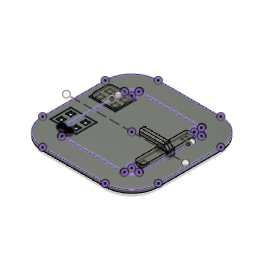
door v4 (Autodesk Fusion 360 design; units mm, degrees)
Autodesk Fusion 360 part; units mm, degrees
sketch "plate" plane through (0, 0, 0) normal (0, 1, 0) x (1, 0, 0)
  line L0 (20, -25) -> (-20, -25)
  line L1 (-25, -20) -> (-25, 20)
  line L2 (-20, 25) -> (20, 25)
  line L3 (25, 20) -> (25, -20)
  line L4 (25, -25) -> (-25, 25) construction
  line L5 (-25, -25) -> (25, 25) construction
  arc A0 (-20, 25) -> (-25, 20) centre (-20, 20) ccw
  arc A1 (-25, -20) -> (-20, -25) centre (-20, -20) ccw
  arc A2 (20, -25) -> (25, -20) centre (20, -20) ccw
  arc A3 (25, 20) -> (20, 25) centre (20, 20) ccw
  line L6 (20, -37) -> (-20, -37)
  arc A4 (-37, -20) -> (-20, -37) centre (-20, -20) ccw
  line L7 (-37, -20) -> (-37, 20)
  arc A5 (-20, 37) -> (-37, 20) centre (-20, 20) ccw
  line L8 (-20, 37) -> (20, 37)
  arc A6 (37, 20) -> (20, 37) centre (20, 20) ccw
  line L9 (37, 20) -> (37, -20)
  arc A7 (20, -37) -> (37, -20) centre (20, -20) ccw
  arc A8 (24.5, 20) -> (20, 24.5) centre (20, 20) ccw
  line L10 (-20, 24.5) -> (20, 24.5)
  arc A9 (-20, 24.5) -> (-24.5, 20) centre (-20, 20) ccw
  line L11 (-24.5, -20) -> (-24.5, 20)
  arc A10 (-24.5, -20) -> (-20, -24.5) centre (-20, -20) ccw
  line L12 (20, -24.5) -> (-20, -24.5)
  arc A11 (20, -24.5) -> (24.5, -20) centre (20, -20) ccw
  line L13 (24.5, 20) -> (24.5, -20)
  dimension "d1" = 50
  dimension "d2" = 50
  dimension "d3" = -12
  dimension "d4" = 5
  dimension "d5" = 0.5
  constraint horizontal L0
  constraint perpendicular L0 L1
  constraint parallel L0 L2
  constraint parallel L1 L3
  constraint coincident L4 origin
  constraint coincident L5 origin
  constraint coincident L4.end L2
  constraint coincident L4.end L1
  constraint tangent L2 A0
  constraint tangent L1 A0
  constraint coincident L5.start L1
  constraint coincident L5.start L0
  constraint tangent L1 A1
  constraint tangent L0 A1
  constraint equal A0 A1
  constraint coincident L4.start L0
  constraint coincident L4.start L3
  constraint tangent L0 A2
  constraint tangent L3 A2
  constraint equal A0 A2
  constraint coincident L5.end L3
  constraint coincident L5.end L2
  constraint tangent L3 A3
  constraint tangent L2 A3
  constraint equal A0 A3
  measures "d1" distance of L4.end L5.end
  measures "d2" distance of L5.start L4.end
  measures "d4" radius of A0
extrude "Extrude1" add sketch "plate" against normal blind 2 makes body 1 at (29, 0, -6.6667) makes body 2 at (-8.1667, 0, -9.6667)
sketch "hinge" plane through (0, 0, 0) normal (0, 1, 0) x (1, 0, 0)
  line L0 (-20, -25) -> (20, -25)
  arc A0 (-25, -20) -> (-20, -25) centre (-20, -20) ccw
  line L1 (-25, 20) -> (-25, -20)
  arc A1 (-20, 25) -> (-25, 20) centre (-20, 20) ccw
  line L2 (20, 25) -> (-20, 25)
  arc A2 (25, 20) -> (20, 25) centre (20, 20) ccw
  line L3 (25, -20) -> (25, 20)
  arc A3 (20, -25) -> (25, -20) centre (20, -20) ccw
  line L4 (20, -37) -> (-20, -37)
  arc A4 (20, -37) -> (37, -20) centre (20, -20) ccw
  line L5 (37, 20) -> (37, -20)
  arc A5 (37, 20) -> (20, 37) centre (20, 20) ccw
  line L6 (-20, 37) -> (20, 37)
  arc A6 (-20, 37) -> (-37, 20) centre (-20, 20) ccw
  line L7 (-37, -20) -> (-37, 20)
  arc A7 (-37, -20) -> (-20, -37) centre (-20, -20) ccw
  line L8 (-24.5, -20) -> (-24.5, 20)
  arc A8 (-24.5, -20) -> (-20, -24.5) centre (-20, -20) ccw
  line L9 (20, -24.5) -> (-20, -24.5)
  arc A9 (20, -24.5) -> (24.5, -20) centre (20, -20) ccw
  line L10 (24.5, 20) -> (24.5, -20)
  arc A10 (24.5, 20) -> (20, 24.5) centre (20, 20) ccw
  line L11 (-20, 24.5) -> (20, 24.5)
  arc A11 (-20, 24.5) -> (-24.5, 20) centre (-20, 20) ccw
  line L12 (-31, 17) -> (-28, 17)
  line L13 (-28, 17) -> (-28, 14)
  line L14 (-28, 14) -> (-31, 14)
  line L15 (-31, 14) -> (-31, 17)
  line L16 (-31, 11) -> (-28, 11)
  line L17 (-28, 11) -> (-28, 8)
  line L18 (-28, 8) -> (-31, 8)
  line L19 (-31, 8) -> (-31, 11)
  line L20 (0, 0) -> (-41.7851, 0) construction
  line L21 (-25, 11.8799) -> (-24.5, 11.8799) construction
  line L22 (-24.75, 11.8799) -> (-24.75, 16.1547) construction
  line L23 (-18.5, 17) -> (-21.5, 17)
  line L24 (-18.5, 14) -> (-18.5, 17)
  line L25 (-21.5, 17) -> (-21.5, 14)
  line L26 (-21.5, 14) -> (-18.5, 14)
  line L27 (-18.5, 11) -> (-21.5, 11)
  line L28 (-18.5, 8) -> (-18.5, 11)
  line L29 (-21.5, 11) -> (-21.5, 8)
  line L30 (-21.5, 8) -> (-18.5, 8)
  line L31 (-33, 19) -> (-16.5, 19)
  line L32 (-16.5, 19) -> (-16.5, 6)
  line L33 (-16.5, 6) -> (-33, 6)
  line L34 (-33, 6) -> (-33, 19)
  line L35 (-18.5, -11) -> (-21.5, -11)
  line L36 (-21.5, -8) -> (-18.5, -8)
  line L37 (-18.5, -17) -> (-21.5, -17)
  line L38 (-31, -8) -> (-31, -11)
  line L39 (-33, -6) -> (-33, -19)
  line L40 (-21.5, -11) -> (-21.5, -8)
  line L41 (-31, -17) -> (-28, -17)
  line L42 (-31, -11) -> (-28, -11)
  line L43 (-18.5, -14) -> (-18.5, -17)
  line L44 (-16.5, -19) -> (-16.5, -6)
  line L45 (-18.5, -8) -> (-18.5, -11)
  line L46 (-28, -17) -> (-28, -14)
  line L47 (-21.5, -17) -> (-21.5, -14)
  line L48 (-21.5, -14) -> (-18.5, -14)
  line L49 (-28, -14) -> (-31, -14)
  line L50 (-16.5, -6) -> (-33, -6)
  line L51 (-33, -19) -> (-16.5, -19)
  line L52 (-31, -14) -> (-31, -17)
  line L53 (-28, -8) -> (-31, -8)
  line L54 (-28, -11) -> (-28, -8)
  line L55 (19.75, 15) -> (22.75, 15)
  line L56 (22.75, 15) -> (22.75, 12)
  line L57 (22.75, 12) -> (19.75, 12)
  line L58 (19.75, 12) -> (19.75, 15)
  line L59 (24.5, 11.146) -> (25, 11.146) construction
  line L60 (24.75, 11.146) -> (24.75, 13.5187) construction
  line L61 (0, 0) -> (34.3439, 0) construction
  line L62 (18.25, 17) -> (24.25, 17)
  line L63 (24.25, 17) -> (24.25, 0)
  line L64 (24.25, 0) -> (18.25, 0)
  line L65 (18.25, 0) -> (18.25, 17)
  line L66 (22.75, -12) -> (19.75, -12)
  line L67 (19.75, -12) -> (19.75, -15)
  line L68 (19.75, -15) -> (22.75, -15)
  line L69 (22.75, -15) -> (22.75, -12)
  line L70 (18.25, -17) -> (24.25, -17)
  line L71 (24.25, -17) -> (24.25, 0)
  line L72 (18.25, 0) -> (18.25, -17)
  point P0 (-25, -20)
  point P1 (-20, -20)
  point P2 (-20, -20)
  point P3 (-24.5, -20)
  dimension "d8" = 3
  dimension "d9" = 3
  dimension "d10" = 3
  dimension "d11" = 3
  dimension "d12" = 3
  dimension "d13" = 3
  dimension "d14" = 8
  dimension "d15" = 2
  dimension "d16" = 2
  dimension "d17" = 2
  dimension "d18" = 2
  dimension "d29" = 3
  dimension "d30" = 3
  dimension "d31" = 2
  dimension "d32" = 12
  dimension "d33" = 1.5
  dimension "d34" = 2
  dimension "d35" = 1.5
  constraint horizontal L12
  constraint vertical L13
  constraint horizontal L14
  constraint vertical L15
  constraint horizontal L16
  constraint vertical L17
  constraint horizontal L18
  constraint vertical L19
  constraint coincident L20.start L61.start
  constraint perpendicular L7 L20
  constraint collinear L13 L17
  constraint coincident L1 L21.start
  constraint coincident L8 L21.end
  constraint perpendicular L8 L21
  constraint midpoint L21 L22.start
  constraint perpendicular L21 L22
  constraint symmetric L12.start L22 L23.start
  constraint symmetric L12.end L22 L23.end
  constraint symmetric L13.end L22 L25.end
  constraint symmetric L14.end L22 L24.start
  constraint symmetric L16.start L22 L27.start
  constraint symmetric L16.end L22 L27.end
  constraint symmetric L17.end L22 L29.end
  constraint symmetric L18.end L22 L28.start
  constraint horizontal L31
  constraint vertical L32
  constraint horizontal L33
  constraint vertical L34
  constraint symmetric L1.start L20 P0
  constraint symmetric A1.centre L20 P2
  constraint symmetric L8.end L20 P3
  constraint symmetric L12.start L20 L41.start
  constraint symmetric L12.end L20 L41.end
  constraint symmetric L13.end L20 L46.end
  constraint symmetric L14.end L20 L49.end
  constraint symmetric L16.start L20 L38.end
  constraint symmetric L16.end L20 L42.end
  constraint symmetric L17.end L20 L53.start
  constraint symmetric L18.end L20 L38.start
  constraint symmetric L20 L23.start L37.start
  constraint symmetric L20 L23.end L37.end
  constraint symmetric L20 L24.start L43.start
  constraint symmetric L20 L25.end L47.end
  constraint symmetric L20 L27.start L35.start
  constraint symmetric L20 L27.end L35.end
  constraint symmetric L20 L28.start L36.end
  constraint symmetric L20 L29.end L36.start
  constraint symmetric L20 L31.start L39.end
  constraint symmetric L20 L31.end L44.start
  constraint symmetric L20 L32.end L44.end
  constraint symmetric L20 L33.end L39.start
  constraint horizontal L55
  constraint vertical L56
  constraint horizontal L57
  constraint vertical L58
  constraint coincident L10 L59.start
  constraint coincident L3 L59.end
  constraint perpendicular L3 L59
  constraint midpoint L59 L60.start
  constraint perpendicular L59 L60
  constraint parallel L20 L61
  constraint horizontal L62
  constraint vertical L63
  constraint horizontal L64
  constraint vertical L65
  constraint collinear L61 L64
  constraint symmetric L55.start L61 L67.end
  constraint symmetric L55.end L61 L68.end
  constraint symmetric L56.end L61 L66.start
  constraint symmetric L57.end L61 L66.end
  constraint symmetric L61 L62.start L70.start
  constraint symmetric L61 L62.end L70.end
  constraint symmetric L61 L63.end L64.start
  constraint symmetric L61 L64.end L65.start
  measures "d8" distance of L12.start L12.end
  measures "d9" distance of L12.start L14.end
  measures "d10" distance of L16.start L16.end
  measures "d11" distance of L16.start L18.end
  measures "d12" distance of L14 L16
  measures "d13" distance of L1 L13
  measures "d14" distance of L18 L20
  measures "d15" distance of L24 L32
  measures "d16" distance of L23 L31
  measures "d17" distance of L30 L33
  measures "d18" distance of L15 L34
  measures "d29" distance of L55.start L55.end
  measures "d30" distance of L55.start L57.end
  measures "d31" distance of L56 L60
  measures "d32" distance of L57 L61
  measures "d33" distance of L58 L65
  measures "d34" distance of L55 L62
  measures "d35" distance of L56 L63
extrude "Extrude2" cut sketch "hinge" against normal blind 3 contours L12 L13 L14 L15 | L16 L17 L18 L19 | L23 L24 L25 L26 | L27 L28 L29 L30 | L35 L36 L40 L45 | L37 L43 L47 L48 | L38 L42 L53 L54 | L41 L46 L49 L52 bodies 1 2
extrude "Extrude3" add sketch "hinge" against normal blind 3 separate body contours L12 L13 L14 L15 | L16 L17 L18 L19 | L23 L24 L25 L26 | L27 L28 L29 L30 makes body 3 at (-21.5, -1, -16) makes body 4 at (-18.5, -1, -9) makes body 5 at (-28, -1, -16) makes body 6 at (-28, -1, -10)
extrude "Extrude4" add sketch "hinge" along normal blind 1 contours L1 L31 L33 L34 | L1 L8 L31 L33 | L8 L31 L32 L33 | L12 L13 L14 L15 | L16 L17 L18 L19 | L23 L24 L25 L26 | L27 L28 L29 L30 bodies 3 4 5 6
fillet "Fillet1" radius 3 4 edges at (-33, 0.5, -6) (-33, 0.5, -19) (-16.5, 0.5, -19) (-16.5, 0.5, -6) on bodies 3
chamfer "Chamfer1" distance 1.5 angle 45 1 edges at (24.5, -2, 0) tangent chain off on bodies 2
chamfer "Chamfer2" distance 1 angle 45 32 edges at (-28, -2, 15.5) (-29.5, -2, 14) (-31, -2, 15.5) (-29.5, -2, 17) (-28, -2, 9.5) (-29.5, -2, 8) (-31, -2, 9.5) (-29.5, -2, 11) (-28, -2, -9.5) (-29.5, -2, -8) (-29.5, -2, -11) (-31, -2, -9.5) (-28, -2, -15.5) (-29.5, -2, -14) (-29.5, -2, -17) (-31, -2, -15.5) (-18.5, -2, 15.5) (-20, -2, 17) (-21.5, -2, 15.5) (-20, -2, 14) (-20, -2, 8) (-21.5, -2, 9.5) (-20, -2, 11) (-18.5, -2, 9.5) (-18.5, -2, -9.5) (-20, -2, -11) (-20, -2, -8) (-21.5, -2, -9.5) (-18.5, -2, -15.5) (-20, -2, -17) (-21.5, -2, -15.5) (-20, -2, -14) tangent chain off on bodies 1 2
extrude "Extrude6" add sketch "hinge" against normal blind 3 separate body contours L55 L56 L57 L58 | L66 L67 L68 L69 makes body 7 at (20.75, -1, -15) makes body 8 at (22.75, -1, 14)
extrude "Extrude7" add sketch "hinge" along normal blind 2 contours L55 L56 L57 L58 | L62 L63 L64 L65 | L64 L70 L71 L72 | L66 L67 L68 L69 bodies 7 8
extrude "Extrude5" cut sketch "hinge" against normal blind 3 contours L55 L56 L57 L58 | L66 L67 L68 L69 bodies 2
fillet "Fillet2" radius 2 4 edges at (18.25, 1, -17) (18.25, 1, 17) (24.25, 1, -17) (24.25, 1, 17) on bodies 7
chamfer "Chamfer3" distance 1 angle 45 6 edges at (21.25, -2, 15) (19.75, -2, 13.5) (21.25, -2, 12) (21.25, -2, -12) (19.75, -2, -13.5) (21.25, -2, -15) tangent chain off on bodies 2
sketch "latch" plane through (0, 0, 0) normal (0, 0, 1) x (1, 0, 0)
  line L0 (-24.5, -2) -> (23, -2)
  line L1 (23, -2) -> (24.5, -0.5)
  line L2 (24.5, -0.5) -> (24.5, 0)
  line L3 (24.5, 0) -> (-24.5, 0)
  line L4 (-24.5, 0) -> (-24.5, -2)
  line L5 (18.25, 0) -> (24.25, 0)
  line L6 (24.25, 2) -> (18.25, 2)
  line L7 (18.25, 2) -> (18.25, 0)
  line L8 (-37, -2) -> (-25, -2)
  line L9 (-25, -2) -> (-25, 0)
  line L10 (-25, 0) -> (-37, 0)
  line L11 (-37, 0) -> (-37, -2)
  line L12 (25, -2) -> (37, -2)
  line L13 (37, -2) -> (37, 0)
  line L14 (37, 0) -> (25, 0)
  line L15 (25, 0) -> (25, -2)
  line L16 (18.25, 0) -> (18.25, -4)
  line L17 (18.25, -4) -> (24.7, -4)
  line L18 (24.7, -4) -> (26.5, -2.2)
  line L19 (26.5, -2.2) -> (23.6223, -2.2)
  line L20 (24.25, 0) -> (24.25, -2.2)
  line L21 (24.25, 0.2) -> (26, 0.2)
  line L22 (26, 0.2) -> (26, 2)
  line L23 (26, 2) -> (24.25, 2)
  line L24 (0, 0) -> (34.3439, 0)
  line L25 (26, 2) -> (6, 2)
  line L26 (6, 2) -> (6, 6)
  line L27 (6, 6) -> (26, 6)
  line L28 (26, 6) -> (26, 2)
  line L29 (24.25, 0) -> (24.25, 2)
  dimension "d45" = 135
  dimension "d46" = 1.5
  dimension "d47" = 2
  dimension "d48" = 0.2
  dimension "d49" = 0.2
  dimension "d50" = 1
  dimension "d51" = 20
  dimension "d52" = 4
  constraint coincident L5.start L7.end
  constraint perpendicular L5 L16
  constraint perpendicular L16 L17
  constraint parallel L0 L19
  constraint coincident L5.end L20.start
  constraint coincident L19 L20.end
  constraint perpendicular L19 L20
  constraint perpendicular L6 L22
  constraint coincident L6.start L23.end
  constraint horizontal L25
  constraint vertical L26
  constraint horizontal L27
  constraint vertical L28
  constraint coincident L21.start L29
  measures "d45" angle of L17 L18
  measures "d46" distance of L15 L18.end
  measures "d47" distance of L0 L17
  measures "d48" distance of L12 L19
  measures "d49" distance of L21 L24
  measures "d50" distance of L15 L22
  measures "d51" distance of L22.end L25.end
  measures "d52" distance of L22.end L27.end
extrude "Extrude8" add sketch "latch" along normal mid plane 4 contours L0 L1 L3 L5 L16 L20 L24 | L0 L1 L16 L17 L18 L19 L20 | L3 L5 L6 L7 L24 L25 L29 | L6 L23 L25 L26 L27 L28 | L21 L22 L23 L25 L29 bodies 7
chamfer "Chamfer4" distance 3 angle 45 1 edges at (26, 6, 0) tangent chain off on bodies 7
chamfer "Chamfer5" distance 3 angle 45 1 edges at (18.25, -4, 0) tangent chain off on bodies 7
fillet "Fillet3" radius 1 14 edges at (6, 6, 0) (6, 2, 0) (6, 4, 2) (6, 4, -2) (14.5, 6, 2) (14.5, 6, -2) (12.125, 2, 2) (12.125, 2, -2) (23, 6, 0) (24.5, 4.5, 2) (24.5, 4.5, -2) (26, 1.6, -2) (26, 3, 0) (26, 1.6, 2) on bodies 7
sketch "latch clearance" plane through (0, -2, 0) normal (0, -1, 0) x (1, 0, 0)
  line L0 (22.75, -11) -> (22.75, -16)
  line L1 (22.75, -16) -> (18.75, -16)
  line L2 (18.75, -16) -> (18.75, -11)
  line L3 (18.75, -11) -> (22.75, -11)
  line L4 (22.75, 16) -> (22.75, 11)
  line L5 (22.75, 11) -> (18.75, 11)
  line L6 (18.75, 11) -> (18.75, 16)
  line L7 (18.75, 16) -> (22.75, 16)
  line L8 (-17.5, -7) -> (-17.5, -12)
  line L9 (-17.5, -12) -> (-22.5, -12)
  line L10 (-22.5, -12) -> (-22.5, -7)
  line L11 (-22.5, -7) -> (-17.5, -7)
  line L12 (-22.5, 18) -> (-17.5, 18)
  line L13 (-17.5, 18) -> (-17.5, 13)
  line L14 (-17.5, 13) -> (-22.5, 13)
  line L15 (-22.5, 13) -> (-22.5, 18)
  line L16 (23, -23.3541) -> (23, 23.3541)
  arc A0 (23, 23.3541) -> (20, 24.5) centre (20, 20) ccw
  line L17 (20, 24.5) -> (-20, 24.5)
  arc A1 (-20, 24.5) -> (-24.5, 20) centre (-20, 20) ccw
  line L18 (-24.5, 20) -> (-24.5, -20)
  arc A2 (-24.5, -20) -> (-20, -24.5) centre (-20, -20) ccw
  line L19 (-20, -24.5) -> (20, -24.5)
  arc A3 (20, -24.5) -> (23, -23.3541) centre (20, -20) ccw
  line L20 (-17.5, 12) -> (-17.5, 7)
  line L21 (-17.5, 7) -> (-22.5, 7)
  line L22 (-22.5, 7) -> (-22.5, 12)
  line L23 (-22.5, 12) -> (-17.5, 12)
  line L24 (-17.5, -13) -> (-17.5, -18)
  line L25 (-17.5, -18) -> (-22.5, -18)
  line L26 (-22.5, -18) -> (-22.5, -13)
  line L27 (-22.5, -13) -> (-17.5, -13)
  line L28 (21.25, 2) -> (21.25, -2)
  line L29 (21.25, -2) -> (24.7, -2)
  line L30 (24.7, -2) -> (24.7, 2)
  line L31 (24.7, 2) -> (21.25, 2)
  line L32 (21.25, 2) -> (18.25, 2)
  line L33 (18.25, 2) -> (18.25, -2)
  line L34 (18.25, -2) -> (21.25, -2)
  line L35 (21.25, -2) -> (21.25, 2)
  line L36 (26.5, -2) -> (26.5, 2)
  line L37 (26.5, 2) -> (24.7, 2)
  line L38 (24.7, 2) -> (24.7, -2)
  line L39 (24.7, -2) -> (26.5, -2)
extrude "Extrude9" cut sketch "latch clearance" against normal blind 10 contours L16 L28 L29 L31 L35 | L16 L29 L30 L31 L38 | L28 L32 L33 L34 L35 | L30 L36 L37 L38 L39 bodies 2
move_face "OffsetFaces1" offset -2 3 faces at (18.25, -1.3333, 0.6667) (21.9167, -0.6667, -2) (21.9167, -0.6667, 2) on bodies 2
named bodies: "door frame", "door door", "door hinge", "door latch"
